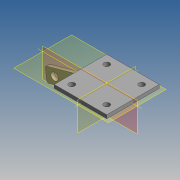
# Autodesk Inventor part: P044_SupportCaméra
Saved by Autodesk Inventor 2021.3 (Build 253353000, 353)
## iProperties
Created: 2022-01-08
Part Number: P044_SupportCaméra
Material: Générique
Document SubType Name: Modeling
Designer: gabri
Density: 1 g/cm^3
Appearance: Par défaut
Author: gabri
Autodesk Inventor part; units mm, degrees
sketch "Sketch2" plane through (0, 0, 0) normal (0, 0, 1) x (1, 0, 0)
  line L0 (30, -30) -> (-30, -30)
  line L1 (-30, -30) -> (-30, 30)
  line L2 (-30, 30) -> (30, 30)
  line L3 (30, 30) -> (30, -30)
  line L4 (30, -30) -> (-30, 30) construction
  line L5 (-30, -30) -> (30, 30) construction
  circle A0 centre (-20, 20) radius 3.25
  circle A1 centre (20, 20) radius 3.25
  circle A2 centre (-20, -20) radius 3.25
  circle A3 centre (20, -20) radius 3.25
  point P0 (0, 0)
  dimension "d0" = 60
  dimension "d1" = 60
  dimension "d13" = 6.5
  dimension "d14" = 6.5
  dimension "d15" = 6.5
  dimension "d16" = 6.5
  dimension "d17" = 10
  dimension "d19" = 10
  dimension "d20" = 10
  dimension "d21" = 10
  constraints: 12 end point, 4 centre point, 4 point on line, 2 midpoint, 2 parallel, 1 horizontal, 1 perpendicular
  measures "d0" distance of L1.end L2.end
  measures "d1" distance between parallel lines of L0 L2
  measures "d13" diameter of A0
  measures "d14" diameter of A1
  measures "d15" diameter of A2
  measures "d16" diameter of A3
  measures "d17" distance from line of L1 A0.centre
  measures "d19" distance from line of L2 A1.centre
  measures "d20" distance from line of L3 A3.centre
  measures "d21" distance from line of L0 A2.centre
extrude "Extrusion1" add sketch "Sketch2" along normal blind 4
sketch "Sketch5" plane through (0, 0, 0) normal (0, 1, 0) x (-1, 0, 0)
  line L0 (-30, 0) -> (30, 0) construction
  line L1 (30, 0) -> (30, 4) construction
  line L2 (-30, 4) -> (30, 4) construction
  line L3 (-30, 0) -> (-30, 4) construction
  line L4 (88.4744, 0) -> (-49.7457, 0) construction
  line L5 (-30, 0) -> (64.1719, -26.056)
  line L6 (66.687, -24.3976) -> (68.3165, -12.3976)
  line L7 (66.868, -10.2009) -> (30, 0)
  line L8 (30, 0) -> (-30, 0)
  arc A0 (68.3165, -12.3976) -> (66.868, -10.2009) centre (66.3347, -12.1284) ccw
  arc A1 (64.1719, -26.056) -> (66.687, -24.3976) centre (64.7052, -24.1284) ccw
  point P0 (66.3789, -26.6667)
  point P1 (68.5516, -10.6667)
  dimension "d26" = 100
  dimension "d31" = 40
  dimension "d32" = 2
  dimension "d37" = 16
  constraints: 8 end point, 4 point on circle, 4 point on line, 4 tangent, 2 centre point, 1 collinear, 1 equal radius, 1 parallel
  measures "d26" distance of L0.start point (66.379, -26.667)
  measures "d31" distance of point (68.552, -10.667) L0.end
  measures "d32" radius of A0
  measures "d37" distance between parallel lines of L5 L7
extrude "Extrusion3" add sketch "Sketch5" along normal mid plane 4
fillet "Fillet1" radius 1 2 edges at (0, 2, 0) (0, -2, 0)
sketch "Sketch6" plane through (0, -2, 0) normal (0, -1, 0) x (1, 0, 0)
  line L0 (-33.6142, -1) -> (26.3858, -1) construction
  line L1 (-33.6142, -1) -> (-66.868, -10.2009) construction
  arc A0 (-66.868, -10.2009) -> (-68.3165, -12.3976) centre (-66.3347, -12.1284) ccw construction
  line L2 (-68.3165, -12.3976) -> (-66.687, -24.3976) construction
  arc A1 (-66.687, -24.3976) -> (-64.1719, -26.056) centre (-64.7052, -24.1284) ccw construction
  line L3 (-64.1719, -26.056) -> (26.3858, -1) construction
  point P0 (0, 0)
  point P1 (-57.7389, -15.9755)
  dimension "d34" = 16
  dimension "d35" = 8
  dimension "d36" = 10
  measures "d34" distance between parallel lines of L3 L1
  measures "d35" distance from line of L1 point (-57.739, -15.976)
  measures "d36" distance from line of point (-57.739, -15.976) L2
hole "Hole1" at (-57.7389, -2, -15.9755) direction (0, 1, 0) diameter 8.5 depth 10
equation "\"d35\" = 0.5 * d34"
body "Solid1"
